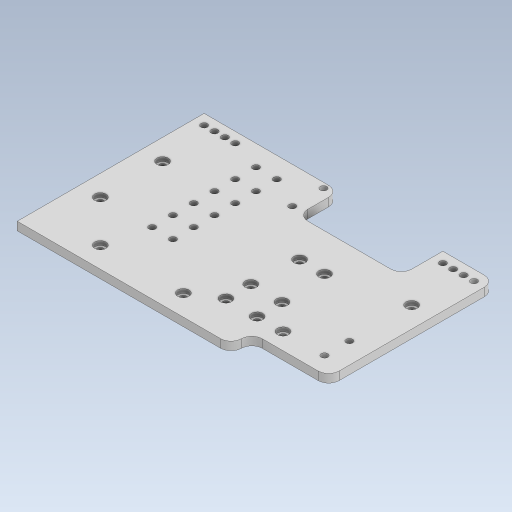
# Autodesk Inventor part: Fix Casis Kanan Belakang
Saved by Autodesk Inventor 2023.5 (Build 275446000, 446)
## iProperties
Created: 2025-10-01
Part Number: Fix Casis Kanan Belakang
Material: Generic
Document SubType Name: Modeling
Designer: Guntur
Density: 1 g/cm^3
Appearance: Default
Author: Guntur
## iProperties of the stored document Fix Casis Kanan Belakang_3DPrint.ipt
Created: 2025-10-18
Part Number: Fix Casis Kanan Belakang_3DPrint
Material: Generic
Document SubType Name: Modeling
Designer: Guntur
Density: 1 g/cm^3
Appearance: Default
Author: Guntur
Autodesk Inventor part; units mm, degrees
ref_plane "YZ Plane" through (0, 0, 0) normal (1, 0, 0) x (0, 1, 0)
ref_plane "XZ Plane" through (0, 0, 0) normal (0, 1, 0) x (-1, 0, 0)
ref_plane "XY Plane" through (0, 0, 0) normal (0, 0, 1) x (1, 0, 0)
sketch "Sketch1" plane through (0, 0, 0) normal (0, 1, 0) x (-1, 0, 0)
  circle A0 centre (-84, -52) radius 1.6
  circle A1 centre (-84, -52) radius 2.75
  circle A2 centre (-82.5, -30) radius 2.75
  line L0 (-70, 0) -> (-70, -90) construction
  line L1 (-65, -70) -> (-115, -70)
  line L2 (-115, -90) -> (-65, -90)
  line L3 (-65, -90) -> (-65, -70)
  line L4 (0, 0) -> (-140, 0)
  line L5 (0, -45) -> (-140, -45) construction
  line L6 (-140, -90) -> (0, -90)
  circle A3 centre (-10, -60) radius 1.6
  circle A4 centre (-82.5, -30) radius 1.6
  circle A5 centre (-130, -60) radius 2.75
  circle A6 centre (-120, -85) radius 1.6
  circle A7 centre (-125, -85) radius 1.6
  circle A8 centre (-130, -60) radius 1.6
  circle A9 centre (-82.5, -18) radius 2.75
  circle A10 centre (-82.5, -18) radius 1.6
  circle A11 centre (-97.5, -18) radius 1.6
  circle A12 centre (-97.5, -18) radius 2.75
  circle A13 centre (-70, -10) radius 1.6
  circle A14 centre (-70, -10) radius 2.75
  circle A15 centre (-96, -52) radius 1.6
  circle A16 centre (-96, -52) radius 2.75
  circle A17 centre (-97.5, -30) radius 1.6
  circle A18 centre (-97.5, -30) radius 2.75
  line L7 (-140, 0) -> (-140, -90)
  circle A19 centre (-130, -30) radius 1.6
  circle A20 centre (-130, -30) radius 2.75
  circle A21 centre (-110, -10) radius 1.6
  circle A22 centre (-120, -5) radius 1.6
  circle A23 centre (-125, -5) radius 1.6
  circle A24 centre (-130, -5) radius 1.6
  circle A25 centre (-135, -5) radius 1.6
  circle A26 centre (-110, -10) radius 2.75
  circle A27 centre (-20, -85) radius 1.6
  circle A28 centre (-10, -60) radius 2.75
  circle A29 centre (-15, -85) radius 1.6
  circle A30 centre (-10, -85) radius 1.6
  circle A31 centre (-5, -85) radius 1.6
  line L8 (0, -90) -> (0, 0)
  circle A32 centre (-10, -30) radius 1.6
  circle A33 centre (-10, -30) radius 2.75
  circle A34 centre (-30, -10) radius 1.6
  circle A35 centre (-30, -10) radius 2.75
  line L9 (-115, -70) -> (-115, -90)
  circle A36 centre (-135, -85) radius 1.6
  circle A37 centre (-130, -85) radius 1.6
  circle A38 centre (-60, -87.5) radius 1.6
  circle A39 centre (-60, -72.5) radius 1.6
  circle A40 centre (-45, -80) radius 1.6
  circle A41 centre (-35, -80) radius 1.6
  circle A42 centre (-35, -70) radius 1.6
  circle A43 centre (-45, -70) radius 1.6
  line L10 (-45, -65) -> (-34, -65)
  circle A44 centre (-35, -50) radius 1.6
  circle A45 centre (-35, -60) radius 1.6
  circle A46 centre (-45, -50) radius 1.6
  circle A47 centre (-45, -60) radius 1.6
  line L11 (-45, -45) -> (-35, -45)
  circle A48 centre (-45, -40) radius 1.6
  circle A49 centre (-35, -40) radius 1.6
  circle A50 centre (-35, -30) radius 1.6
  circle A51 centre (-45, -30) radius 1.6
  circle A52 centre (-115, -5) radius 1.65
  circle A53 centre (-110, -18) radius 1.6
  circle A54 centre (-110, -18) radius 2.75
  circle A55 centre (-130, -10) radius 1.6
  circle A56 centre (-130, -18) radius 1.6
  circle A57 centre (-130, -10) radius 2.75
  circle A58 centre (-130, -18) radius 2.75
  line L12 (-140, 0) -> (-103, 0)
  line L13 (-103, 0) -> (-103, -10)
  line L14 (-103, -10) -> (-140, -10)
  line L15 (-140, -10) -> (-140, 0)
  point P0 (-66.6052, -46.0515)
  point P1 (-140, -10)
  point P2 (-131.6, -10)
  point P3 (-132.75, -10)
  point P4 (-127.25, -10)
  point P5 (-128.4, -10)
  point P6 (-112.75, -10)
  point P7 (-107.25, -10)
  point P8 (-111.6, -10)
  point P9 (-108.4, -10)
  dimension "d12" = 140
  dimension "d13" = 90
  dimension "d14" = 10
  dimension "d15" = 10
  dimension "d16" = 10
  dimension "d17" = 10
  dimension "d18" = 10
  dimension "d19" = 10
  dimension "d20" = 10
  dimension "d21" = 3.2
  dimension "d22" = 2.5
  dimension "d23" = 5
  dimension "d24" = 3.2
  dimension "d25" = 15
  dimension "d26" = 3.2
  dimension "d27" = 3.2
  dimension "d28" = 10
  dimension "d29" = 3.2
  dimension "d30" = 10
  dimension "d31" = 3.2
  dimension "d32" = 10
  dimension "d33" = 10
  dimension "d35" = 5
  dimension "d36" = 25
  dimension "d37" = 3.3
  dimension "d38" = 5
  dimension "d40" = 3.2
  dimension "d41" = 5.5
  dimension "d42" = 3.2
  dimension "d43" = 3.2
  dimension "d44" = 5.5
  dimension "d45" = 5.5
  dimension "d46" = 10
  constraints: 59 centre point, 32 end point, 16 coincident, 8 symmetric about line, 3 horizontal, 3 point on line, 2 parallel, 1 perpendicular, 8 other
  measures "d12" distance of L4.start L4.end
  measures "d13" distance of L6.end L4.start
  measures "d14" distance from line of L8 A33.centre
  measures "d15" distance from line of L8 A3.centre
  measures "d16" distance from line of L4 A34.centre
  measures "d17" distance from line of L4 A14.centre
  measures "d18" distance from line of L4 A21.centre
  measures "d19" distance from line of L7 A20.centre
  measures "d20" distance from line of L7 A5.centre
  measures "d21" diameter of A38
  measures "d22" distance from line of L6 A38.centre
  measures "d23" distance from line of L3 A38.centre
  measures "d24" diameter of A39
  measures "d25" distance of A38.centre A39.centre
  measures "d26" diameter of A43
  measures "d27" diameter of A40
  measures "d28" distance of A40.centre A43.centre
  measures "d29" diameter of A41
  measures "d30" distance of A40.centre A41.centre
  measures "d31" diameter of A42
  measures "d32" distance of A43.centre A42.centre
  measures "d33" distance from line of L6 A40.centre
  measures "d35" distance from line of L10 A43.centre
  measures "d36" distance from line of L11 A43.centre
  measures "d37" diameter of A52
  measures "d38" distance of A22.centre A52.centre
  measures "d40" diameter of A53
  measures "d41" diameter of A54
  measures "d42" diameter of A55
  measures "d43" diameter of A56
  measures "d44" diameter of A57
  measures "d45" diameter of A58
  measures "d46" distance of L12.end L13.end
extrude "Extrusion1" add sketch "Sketch1" along normal blind 4 contours L1 L9 L6 L7 L14 A57 A26 L13 L4 L8 L3 | L14 A55 A57 | L14 A55 | A26 L14 A21 | A21 L14 | A20 | A58 picked at (-132.3245, -10.347) picked at (-130.4722, -10.2479) picked at (-112.3245, -10.347) picked at (-110.4603, -10.6015)
extrude "Extrusion2" add sketch "Sketch1" along normal blind 2 contours A1 | A2 | A26 L14 A21 | A5 | A9 | A12 | A14 | A16 | A18 | A20 | A28 | A33 | A35 | A54 picked at (-112.3245, -10.347)
fillet "Fillet1" radius 5 7 edges at (65, 2, -90) (65, 2, -70) (115, 2, -70) (140, 2, -90) (103, 2, 0) (103, 2, -10) (140, 2, -10)
body "Solid1"
